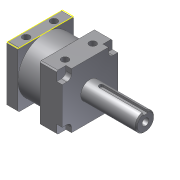
# Autodesk Inventor part: P60Gearbox_1stage
Saved by Autodesk Inventor 2012 (Build 160160000, 160)
## iProperties
Created: 2012-01-17
Part Number: P60Gearbox_1stage
Material: Default
Document SubType Name: Modeling
Designer: JesseK
Density: 1 g/cm^3
Mass: 49.4018 g
Surface Area: 130.896 cm^2
Volume: 49.4018 cm^3
Author: JesseK
Autodesk Inventor part; units mm, degrees
ref_plane "YZ Plane" through (0, 0, 0) normal (1, 0, 0) x (0, 1, 0)
ref_plane "XZ Plane" through (0, 0, 0) normal (0, 1, 0) x (-1, 0, 0)
ref_plane "XY Plane" through (0, 0, 0) normal (0, 0, 1) x (1, 0, 0)
sketch "Sketch1" plane through (0, 0, 0) normal (0, 0, 1) x (1, 0, 0)
  line L0 (0, 0) -> (7.62, 0)
  line L1 (7.62, 0) -> (7.62, 38.1)
  line L2 (7.62, 38.1) -> (0, 38.1)
  line L3 (0, 38.1) -> (0, 0)
  dimension "d0" = 7.62
  dimension "d1" = 38.1
  constraints: 8 end point, 2 parallel, 1 horizontal, 1 perpendicular
  measures "d0" distance of L1.end L2.end
  measures "d1" distance of L2.end L0.start
extrude "Extrusion1" add sketch "Sketch1" along normal blind 38.1
sketch "Sketch2" plane through (7.62, 0, 0) normal (1, 0, 0) x (0, 0, -1)
  line L0 (-38.1, 38.1) -> (-38.1, 0) projected
  line L1 (0, 38.1) -> (-38.1, 38.1) projected
  circle A0 centre (-19.05, 19.05) radius 19.05
  dimension "d4" = 38.1
  dimension "d5" = 19.05
  dimension "d6" = 19.05
  constraints: 1 centre point
  measures "d4" diameter of A0
  measures "d5" distance from line of L1 A0.centre
  measures "d6" distance from line of L0 A0.centre
extrude "Extrusion2" add sketch "Sketch2" along normal blind 15.24 contours A0
sketch "Sketch3" plane through (0, 38.1, 0) normal (0, 1, 0) x (1, 0, 0)
  line L0 (0, -38.1) -> (7.62, -38.1) projected
  line L1 (7.62, 0) -> (7.62, -38.1) projected
  line L2 (7.62, 0) -> (0, 0) projected
  line L3 (0, 0) -> (0, -38.1) projected
sketch "Sketch4" plane through (22.86, 19.05, 19.05) normal (1, 0, 0) x (0, 0, -1)
  line L0 (-19.0547, 19.05) -> (19.05, 19.05)
  line L1 (19.05, 19.05) -> (19.05, -19.05)
  line L2 (19.05, -19.05) -> (-19.0547, -19.05)
  line L3 (-19.0547, -19.05) -> (-19.0547, 19.05)
  dimension "d9" = 38.1
  dimension "d10" = 38.1046
  constraints: 8 end point, 2 parallel, 1 horizontal, 1 perpendicular
  measures "d9" distance of L0.end L1.end
  measures "d10" distance of L1.end L2.end
extrude "Extrusion3" add sketch "Sketch4" along normal blind 15.24
sketch "Sketch5" plane through (38.1, 19.05, 19.05) normal (1, 0, 0) x (0, 0, -1)
  line L0 (19.05, -19.05) -> (-19.0547, -19.05) projected
  line L1 (19.05, 19.05) -> (19.05, -19.05) projected
  circle A0 centre (0, 0) radius 6.35
  dimension "d13" = 19.05
  dimension "d14" = 19.05
  dimension "d15" = 12.7
  constraints: 1 centre point
  measures "d13" distance from line of L1 A0.centre
  measures "d14" distance from line of L0 A0.centre
  measures "d15" diameter of A0
extrude "Extrusion4" add sketch "Sketch5" along normal blind 38.1
sketch "Sketch6" plane through (38.1, 19.05, 19.05) normal (1, 0, 0) x (0, 0, -1)
  line L0 (19.05, -19.05) -> (-19.0547, -19.05) projected
  line L1 (19.05, 19.05) -> (19.05, -19.05) projected
  line L2 (-19.0547, 19.05) -> (19.05, 19.05) projected
  line L3 (-19.0547, -19.05) -> (-19.0547, 19.05) projected
  line L4 (-12.7047, 19.05) -> (-12.7047, 15.875)
  line L5 (-15.8797, 12.7) -> (-19.0547, 12.7)
  arc A0 (-15.8797, 12.7) -> (-12.7047, 15.875) centre (-15.8797, 15.875) ccw
  line L6 (-12.7047, 19.05) -> (-19.0547, 19.05)
  line L7 (-19.0547, 19.05) -> (-19.0547, 12.7)
  line L8 (-19.0547, 0) -> (19.05, 0) construction
  line L9 (-0.0023, 19.05) -> (-0.0023, -19.05) construction
  line L10 (12.7, 19.05) -> (12.7, 15.875)
  line L11 (15.875, 12.7) -> (19.05, 12.7)
  arc A1 (12.7, 15.875) -> (15.875, 12.7) centre (15.875, 15.875) ccw
  line L12 (12.7, 19.05) -> (19.05, 19.05)
  line L13 (19.05, 19.05) -> (19.05, 12.7)
  line L14 (-12.7047, -19.05) -> (-12.7047, -15.875)
  line L15 (-15.8797, -12.7) -> (-19.0547, -12.7)
  arc A2 (-12.7047, -15.875) -> (-15.8797, -12.7) centre (-15.8797, -15.875) ccw
  line L16 (-12.7047, -19.05) -> (-19.0547, -19.05)
  line L17 (-19.0547, -19.05) -> (-19.0547, -12.7)
  line L18 (19.05, -19.05) -> (19.05, -12.7)
  line L19 (12.7, -19.05) -> (19.05, -19.05)
  line L20 (12.7, -19.05) -> (12.7, -15.875)
  arc A3 (15.875, -12.7) -> (12.7, -15.875) centre (15.875, -15.875) ccw
  line L21 (15.875, -12.7) -> (19.05, -12.7)
  dimension "d18" = 6.35
  dimension "d19" = 6.35
  dimension "d20" = 3.175
  constraints: 36 end point, 15 symmetric about line, 8 point on circle, 4 centre point, 4 midpoint, 2 horizontal, 2 point on line, 2 tangent, 2 vertical, 3 other
  measures "d18" distance between parallel lines of L3 L4
  measures "d19" distance between parallel lines of L2 L5
  measures "d20" radius of A0
extrude "Extrusion5" cut sketch "Sketch6" against normal blind 3.81 contours L0 L20 A3 L21 L1 | L0 L3 L15 A2 L14 | L11 A1 L10 L2 L1 | L3 L2 L4 A0 L5
sketch "Sketch7" plane through (0, 0, 0) normal (-1, 0, 0) x (0, 0, 1)
  line L0 (38.1, 0) -> (38.1, 38.1) projected
  line L1 (0, 38.1) -> (38.1, 38.1) projected
  circle A0 centre (19.05, 19.05) radius 9.525
  dimension "d23" = 19.05
  dimension "d24" = 19.05
  dimension "d25" = 19.05
  constraints: 1 centre point
  measures "d23" diameter of A0
  measures "d24" distance from line of L1 A0.centre
  measures "d25" distance from line of L0 A0.centre
extrude "Extrusion6" cut sketch "Sketch7" against normal blind 7.62
sketch "Sketch8" plane through (22.86, 38.1, 38.1047) normal (0, 1, 0) x (1, 0, 0)
  line L0 (0, 38.1047) -> (11.43, 38.1047) projected
  line L1 (0, 38.1047) -> (0, 19.0547) projected
  line L2 (0, 19.0547) -> (0, 0) projected
  line L3 (0, 0) -> (11.43, 0) projected
  circle A0 centre (7.62, 28.5797) radius 2.3813
  circle A1 centre (7.62, 9.525) radius 2.3813
  circle A2 centre (-19.05, 9.5297) radius 2.3813
  circle A3 centre (-19.05, 28.5797) radius 2.3813
  line L4 (-15.24, 38.1047) -> (-22.86, 38.1047) projected
  line L5 (-22.86, 0.0047) -> (-15.24, 0.0047) projected
  line L6 (-22.86, 38.1047) -> (-22.86, 0.0047) projected
  dimension "d28" = 4.7625
  dimension "d29" = 9.525
  dimension "d30" = 9.525
  dimension "d31" = 3.81
  dimension "d32" = 3.81
  dimension "d33" = 7.62
  dimension "d34" = 7.62
  dimension "d35" = 9.525
  dimension "d36" = 9.525
  constraints: 4 centre point, 3 equal radius
  measures "d28" diameter of A3
  measures "d29" distance from line of L4 A3.centre
  measures "d30" distance from line of L5 A2.centre
  measures "d31" distance from line of L6 A2.centre
  measures "d32" distance from line of L6 A3.centre
  measures "d33" distance from line of L1 A0.centre
  measures "d34" distance from line of L2 A1.centre
  measures "d35" distance from line of L0 A0.centre
  measures "d36" distance from line of L3 A1.centre
extrude "Extrusion7" cut sketch "Sketch8" against normal through all
sketch "Sketch11" plane through (76.2, 19.05, 19.05) normal (1, 0, 0) x (0, 0, -1)
  circle A0 centre (0, 0) radius 6.35 projected
  line L0 (-1.5875, 6.1484) -> (-1.5875, 4.5609)
  line L1 (-1.5875, 4.5609) -> (1.5875, 4.5609)
  line L2 (1.5875, 4.5609) -> (1.5875, 6.1484)
  arc A1 (1.5875, 6.1484) -> (-1.5875, 6.1484) centre (0, 0) ccw
  point P0 (19.05, -19.05)
  dimension "d48" = 3.175
  dimension "d49" = 1.5875
  constraints: 6 end point, 2 point on circle, 2 vertical, 1 centre point, 1 coincident, 1 horizontal, 1 parallel, 2 other
  measures "d48" distance of L0.end L1.end
  measures "d49" distance of L0.start L0.end
extrude "Extrusion9" cut sketch "Sketch11" against normal blind 31.75 contours L2 L1 L0 A0 picked at (0.1781, 5.1498)
chamfer "Chamfer2" distance 0.7937 angle 45 2 edges at (76.2, 14.0299, 22.9386) (76.2, 22.9386, 14.0299)
sketch "Sketch12" plane through (76.2, 19.05, 19.05) normal (1, 0, 0) x (0, 0, -1)
  arc A0 (-1.5875, 5.3246) -> (1.5875, 5.3246) centre (0, 0) ccw projected
  circle A1 centre (0, 0) radius 2.3813
  point P0 (19.05, -19.05)
  dimension "d55" = 4.7625
  constraints: 1 centre point, 1 coincident
  measures "d55" diameter of A1
extrude "Extrusion10" cut sketch "Sketch12" against normal blind 25.4
fillet "Fillet1" radius 1.5875 2 edges at (44.45, 24.4046, 17.4625) (44.45, 24.4046, 20.6375)
chamfer "Chamfer3" distance 0.7937 angle 45 8 edges at (3.81, 38.1, 38.1) (3.81, 38.1, 0) (28.575, 38.1, 0) (28.575, 38.1, 38.1047) (28.575, 0, 38.1047) (3.81, 0, 38.1) (28.575, 0, 0) (3.81, 0, 0)
body "Solid1"
